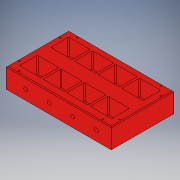
# Autodesk Inventor part: UNLHEP-14-01-P-004_ChuckForGantry
Saved by Autodesk Inventor 2019.4 (Build 234330000, 330)
## iProperties
Created: 2014-01-09
Part Number: UNLHEP-14-01-P-004_ChuckForGantry
Material: Aluminum, Anodized Red
Document SubType Name: Modeling
Designer: Frank Meier
Density: 2.7 g/cm^3
Project: UNL Pixel Phase I
Mass: 2699.72 g
Surface Area: 1115.91 cm^2
Volume: 999.896 cm^3
Appearance: Anodized - Red
Author: Frank Meier
Revision Number: 00
Autodesk Inventor part; units mm, degrees
ref_plane "YZ Plane" through (0, 0, 0) normal (1, 0, 0) x (0, 1, 0)
ref_plane "XZ Plane" through (0, 0, 0) normal (0, 1, 0) x (-1, 0, 0)
ref_plane "XY Plane" through (0, 0, 0) normal (0, 0, 1) x (1, 0, 0)
sketch "Skizze1" plane through (0, 0, 0) normal (0, 0, 1) x (1, 0, 0)
  line L0 (-117.475, -69.85) -> (117.475, -69.85)
  line L1 (117.475, -69.85) -> (117.475, 69.85)
  line L2 (117.475, 69.85) -> (-117.475, 69.85)
  line L3 (-117.475, 69.85) -> (-117.475, -69.85)
  line L4 (-117.475, -69.85) -> (117.475, 69.85) construction
  line L5 (117.475, -69.85) -> (-117.475, 69.85) construction
  point P0 (0, 0)
  dimension "d0" = 234.95
  dimension "d2" = 139.7
  constraints: 12 end point, 2 midpoint, 2 parallel, 1 horizontal, 1 perpendicular
  measures "d0" distance of L1.end L2.end
  measures "d2" distance of L0.end L1.end
extrude "Extrusion1" add sketch "Skizze1" along normal blind 44.45
chamfer "Fase1" distance 2 angle 45 4 edges at (0, -69.85, 44.45) (-117.475, 0, 44.45) (0, 69.85, 44.45) (117.475, 0, 44.45)
sketch "Skizze4" plane through (0, 0, 44.45) normal (0, 0, 1) x (1, 0, 0)
  line L0 (117.475, 69.85) -> (-117.475, 69.85) projected
  line L1 (117.475, -69.85) -> (117.475, 69.85) projected
  line L2 (-117.475, 69.85) -> (-117.475, -69.85) projected
  line L3 (-117.475, -69.85) -> (117.475, -69.85) projected
  point P0 (-112.475, 45.85)
  point P1 (-112.475, -45.85)
  point P2 (-93.475, -64.85)
  point P3 (-93.475, 64.85)
  point P4 (93.475, 64.85)
  point P5 (112.475, 45.85)
  point P6 (112.475, -45.85)
  point P7 (93.475, -64.85)
  dimension "d153" = 24
  dimension "d154" = 24
  dimension "d155" = 5
  dimension "d156" = 5
  dimension "d157" = 24
  dimension "d158" = 5
  dimension "d159" = 5
  dimension "d160" = 24
  dimension "d161" = 24
  dimension "d162" = 5
  dimension "d163" = 5
  dimension "d164" = 24
  dimension "d165" = 5
  dimension "d166" = 24
  dimension "d167" = 5
  dimension "d168" = 24
  measures "d153" distance from line of L0 point (-112.475, 45.85)
  measures "d154" distance from line of L3 point (-112.475, -45.85)
  measures "d155" distance from line of L2 point (-112.475, -45.85)
  measures "d156" distance from line of L3 point (-93.475, -64.85)
  measures "d157" distance from line of L2 point (-93.475, -64.85)
  measures "d158" distance from line of L2 point (-112.475, 45.85)
  measures "d159" distance from line of L0 point (-93.475, 64.85)
  measures "d160" distance from line of L2 point (-93.475, 64.85)
  measures "d161" distance from line of L1 point (93.475, 64.85)
  measures "d162" distance from line of L0 point (93.475, 64.85)
  measures "d163" distance from line of L1 point (112.475, 45.85)
  measures "d164" distance from line of L0 point (112.475, 45.85)
  measures "d165" distance from line of L1 point (112.475, -45.85)
  measures "d166" distance from line of L3 point (112.475, -45.85)
  measures "d167" distance from line of L3 point (93.475, -64.85)
  measures "d168" distance from line of L1 point (93.475, -64.85)
hole "Bohrung7" at (-112.475, 45.85, 44.45) at (-112.475, -45.85, 44.45) at (-93.475, -64.85, 44.45) at (-93.475, 64.85, 44.45) at (93.475, 64.85, 44.45) at (112.475, 45.85, 44.45) at (112.475, -45.85, 44.45) at (93.475, -64.85, 44.45) direction (0, 0, -1) diameter 3.242 depth 20 tip angle 118 thread size "M4x0.7" class "6H" standard "ISO Metric profile"
sketch "Sketch12" plane through (0, 0, 44.45) normal (0, 0, 1) x (1, 0, 0)
  line L0 (-101.975, 56.35) -> (-58.225, 56.35)
  line L1 (-56.225, 54.35) -> (-56.225, 18.35)
  line L2 (-58.225, 16.35) -> (-101.975, 16.35)
  line L3 (-103.975, 18.35) -> (-103.975, 54.35)
  circle A0 centre (-112.475, 45.85) radius 1.621 projected
  circle A1 centre (-112.475, 45.85) radius 1.621 projected
  circle A2 centre (-93.475, 64.85) radius 1.621 projected
  arc A3 (-101.975, 56.35) -> (-103.975, 54.35) centre (-101.975, 54.35) ccw
  arc A4 (-56.225, 54.35) -> (-58.225, 56.35) centre (-58.225, 54.35) ccw
  arc A5 (-58.225, 16.35) -> (-56.225, 18.35) centre (-58.225, 18.35) ccw
  arc A6 (-103.975, 18.35) -> (-101.975, 16.35) centre (-101.975, 18.35) ccw
  arc A7 (-49.225, 56.35) -> (-51.225, 54.35) centre (-49.225, 54.35) ccw
  line L4 (-51.225, 18.35) -> (-51.225, 54.35)
  line L5 (-49.225, 56.35) -> (-5.475, 56.35)
  arc A8 (-3.475, 54.35) -> (-5.475, 56.35) centre (-5.475, 54.35) ccw
  line L6 (-3.475, 54.35) -> (-3.475, 18.35)
  arc A9 (-5.475, 16.35) -> (-3.475, 18.35) centre (-5.475, 18.35) ccw
  line L7 (-5.475, 16.35) -> (-49.225, 16.35)
  arc A10 (-51.225, 18.35) -> (-49.225, 16.35) centre (-49.225, 18.35) ccw
  arc A11 (3.525, 56.35) -> (1.525, 54.35) centre (3.525, 54.35) ccw
  line L8 (1.525, 18.35) -> (1.525, 54.35)
  line L9 (3.525, 56.35) -> (47.275, 56.35)
  arc A12 (49.275, 54.35) -> (47.275, 56.35) centre (47.275, 54.35) ccw
  line L10 (49.275, 54.35) -> (49.275, 18.35)
  arc A13 (47.275, 16.35) -> (49.275, 18.35) centre (47.275, 18.35) ccw
  line L11 (47.275, 16.35) -> (3.525, 16.35)
  arc A14 (1.525, 18.35) -> (3.525, 16.35) centre (3.525, 18.35) ccw
  arc A15 (56.275, 56.35) -> (54.275, 54.35) centre (56.275, 54.35) ccw
  line L12 (54.275, 18.35) -> (54.275, 54.35)
  line L13 (56.275, 56.35) -> (100.025, 56.35)
  arc A16 (102.025, 54.35) -> (100.025, 56.35) centre (100.025, 54.35) ccw
  line L14 (102.025, 54.35) -> (102.025, 18.35)
  arc A17 (100.025, 16.35) -> (102.025, 18.35) centre (100.025, 18.35) ccw
  line L15 (100.025, 16.35) -> (56.275, 16.35)
  arc A18 (54.275, 18.35) -> (56.275, 16.35) centre (56.275, 18.35) ccw
  arc A19 (-101.975, -13.65) -> (-103.975, -15.65) centre (-101.975, -15.65) ccw
  line L16 (-103.975, -51.65) -> (-103.975, -15.65)
  line L17 (-101.975, -13.65) -> (-58.225, -13.65)
  arc A20 (-56.225, -15.65) -> (-58.225, -13.65) centre (-58.225, -15.65) ccw
  line L18 (-56.225, -15.65) -> (-56.225, -51.65)
  arc A21 (-58.225, -53.65) -> (-56.225, -51.65) centre (-58.225, -51.65) ccw
  line L19 (-58.225, -53.65) -> (-101.975, -53.65)
  arc A22 (-103.975, -51.65) -> (-101.975, -53.65) centre (-101.975, -51.65) ccw
  arc A23 (-49.225, -13.65) -> (-51.225, -15.65) centre (-49.225, -15.65) ccw
  line L20 (-51.225, -51.65) -> (-51.225, -15.65)
  line L21 (-49.225, -13.65) -> (-5.475, -13.65)
  arc A24 (-3.475, -15.65) -> (-5.475, -13.65) centre (-5.475, -15.65) ccw
  line L22 (-3.475, -15.65) -> (-3.475, -51.65)
  arc A25 (-5.475, -53.65) -> (-3.475, -51.65) centre (-5.475, -51.65) ccw
  line L23 (-5.475, -53.65) -> (-49.225, -53.65)
  arc A26 (-51.225, -51.65) -> (-49.225, -53.65) centre (-49.225, -51.65) ccw
  arc A27 (3.525, -13.65) -> (1.525, -15.65) centre (3.525, -15.65) ccw
  line L24 (1.525, -51.65) -> (1.525, -15.65)
  line L25 (3.525, -13.65) -> (47.275, -13.65)
  arc A28 (49.275, -15.65) -> (47.275, -13.65) centre (47.275, -15.65) ccw
  line L26 (49.275, -15.65) -> (49.275, -51.65)
  arc A29 (47.275, -53.65) -> (49.275, -51.65) centre (47.275, -51.65) ccw
  line L27 (47.275, -53.65) -> (3.525, -53.65)
  arc A30 (1.525, -51.65) -> (3.525, -53.65) centre (3.525, -51.65) ccw
  arc A31 (56.275, -13.65) -> (54.275, -15.65) centre (56.275, -15.65) ccw
  line L28 (54.275, -51.65) -> (54.275, -15.65)
  line L29 (56.275, -13.65) -> (100.025, -13.65)
  arc A32 (102.025, -15.65) -> (100.025, -13.65) centre (100.025, -15.65) ccw
  line L30 (102.025, -15.65) -> (102.025, -51.65)
  arc A33 (100.025, -53.65) -> (102.025, -51.65) centre (100.025, -51.65) ccw
  line L31 (100.025, -53.65) -> (56.275, -53.65)
  arc A34 (54.275, -51.65) -> (56.275, -53.65) centre (56.275, -51.65) ccw
  point P0 (0, 0)
  point P1 (-56.225, 16.35)
  point P2 (-56.225, 56.35)
  point P3 (-103.975, 16.35)
  point P4 (-51.225, 16.35)
  point P5 (-3.475, 56.35)
  point P6 (-3.475, 16.35)
  point P7 (1.525, 16.35)
  point P8 (49.275, 56.35)
  point P9 (49.275, 16.35)
  point P10 (54.275, 16.35)
  point P11 (102.025, 56.35)
  point P12 (102.025, 16.35)
  point P13 (-103.975, -53.65)
  point P14 (-56.225, -13.65)
  point P15 (-56.225, -53.65)
  point P16 (-51.225, -53.65)
  point P17 (-3.475, -13.65)
  point P18 (-3.475, -53.65)
  point P19 (1.525, -53.65)
  point P20 (49.275, -13.65)
  point P21 (49.275, -53.65)
  point P22 (54.275, -53.65)
  point P23 (102.025, -13.65)
  point P24 (102.025, -53.65)
  dimension "d193" = 47.75
  dimension "d194" = 40
  dimension "d195" = 8.5
  dimension "d196" = 8.5
  dimension "d197" = 2
  dimension "d200" = 52.75
  dimension "d203" = 70
  constraints: 64 end point, 64 point on circle, 48 point on line, 32 centre point, 8 tangent, 3 equal radius, 2 collinear, 2 horizontal, 2 parallel, 1 perpendicular, 1 vertical, 159 other
  measures "d193" distance of point (-56.225, 16.35) point (-103.975, 16.35)
  measures "d194" distance of point (-56.225, 56.35) point (-56.225, 16.35)
  measures "d195" distance from line of L3 point (-112.475, 45.85)
  measures "d196" distance from line of L0 point (-93.475, 64.85)
  measures "d197" radius of A3
  measures "d200" distance of L3.end L4.end
  measures "d203" distance of L3.end L16.end
extrude "Extrusion5" cut sketch "Sketch12" against normal blind 36 contours L0 A4 L1 A5 L2 A6 L3 A3 | L5 A8 L6 A9 L7 A10 L4 A7 | L9 A12 L10 A13 L11 A14 L8 A11 | L13 A16 L14 A17 L15 A18 L12 A15 | L17 A20 L18 A21 L19 A22 L16 A19 | L21 A24 L22 A25 L23 A26 L20 A23 | L25 A28 L26 A29 L27 A30 L24 A27 | L29 A32 L30 A33 L31 A34 L28 A31
sketch "Sketch13" plane through (-117.475, -69.85, 0) normal (0, -1, 0) x (1, 0, 0)
  line L0 (232.95, 44.45) -> (2, 44.45) projected
  point P0 (117.475, 0)
  point P1 (43.375, 21.45)
  point P2 (96.125, 21.45)
  point P3 (148.875, 21.45)
  point P4 (201.625, 21.45)
  dimension "d209" = 23
  dimension "d212" = 52.75
  constraints: 1 horizontal, 3 other
  measures "d209" distance from line of point (43.375, 21.45) L0
  measures "d212" distance of point (43.375, 21.45) point (96.125, 21.45)
hole "Hole9" at (-74.1, -69.85, 21.45) at (-21.35, -69.85, 21.45) at (31.4, -69.85, 21.45) at (84.15, -69.85, 21.45) direction (0, 1, 0) diameter 7.95 depth 16.2 tip angle 118 taper from width 8.7366 to width 8.304 over 6.924 thread size "1/8" designation "1/8 - 27 NPT" standard "NPT"
sketch "Sketch14" plane through (-117.475, 69.85, 0) normal (0, 1, 0) x (1, 0, 0)
  circle A0 centre (43.375, -21.45) radius 4.3684 projected
  line L0 (234.95, -42.45) -> (0, -42.45) projected
  point P0 (117.475, 0)
  point P1 (96.125, -21.45)
  point P2 (148.875, -21.45)
  point P3 (201.625, -21.45)
  dimension "d228" = 52.75
  constraints: 1 coincident, 1 horizontal, 3 other
  measures "d228" distance of point (43.375, -21.45) point (96.125, -21.45)
hole "Hole10" at (-74.1, 69.85, 21.45) at (-21.35, 69.85, 21.45) at (31.4, 69.85, 21.45) at (84.15, 69.85, 21.45) direction (0, -1, 0) diameter 7.95 depth 13.5 tip angle 118 taper from width 8.7366 to width 8.304 over 6.924 thread size "1/8" designation "1/8 - 27 NPT" standard "NPT"
sketch "Sketch15" plane through (0, 0, 0) normal (0, 0, -1) x (-1, 0, 0)
  line L0 (117.475, -69.85) -> (-117.475, -69.85) projected
  line L1 (117.475, 69.85) -> (117.475, -69.85) projected
  point P0 (0, 0)
  point P1 (76.2, -25.4)
  point P2 (-76.2, -25.4)
  point P3 (76.2, 25.4)
  point P4 (-76.2, 25.4)
  dimension "d242" = 25.4
  dimension "d243" = 76.2
  dimension "d246" = 152.4
  dimension "d249" = 50.8
  constraints: 1 horizontal, 1 vertical, 3 other
  measures "d242" vertical distance of point (0, 0) point (76.2, -25.4)
  measures "d243" horizontal distance of point (0, 0) point (76.2, -25.4)
  measures "d246" distance of point (76.2, -25.4) point (-76.2, -25.4)
  measures "d249" distance of point (76.2, -25.4) point (76.2, 25.4)
hole "Hole11" at (-76.2, -25.4, 0) at (76.2, -25.4, 0) at (-76.2, 25.4, 0) at (76.2, 25.4, 0) direction (0, 0, 1) diameter 6.756 depth 8.45 tip angle 118 clearance for "Flat Head Machine Screw (82)" size "1/4" standard "Ansi Unified Screw Threads"
